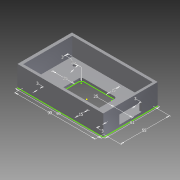
# Autodesk Inventor part: layer line sensor
Saved by Autodesk Inventor 2012 (Build 160160000, 160)
## iProperties
Created: 2012-11-27
Part Number: layer line sensor
Material: Default
Document SubType Name: Modeling
Designer: irwan
Density: 1 g/cm^3
Author: irwan
Autodesk Inventor part; units mm, degrees
ref_plane "YZ Plane" through (0, 0, 0) normal (1, 0, 0) x (0, 1, 0)
ref_plane "XZ Plane" through (0, 0, 0) normal (0, 1, 0) x (-1, 0, 0)
ref_plane "XY Plane" through (0, 0, 0) normal (0, 0, 1) x (1, 0, 0)
sketch "Sketch1" plane through (0, 0, 0) normal (0, 0, 1) x (1, 0, 0)
  line L0 (-50.0201, 33.5227) -> (45.9799, 33.5227)
  line L1 (45.9799, 33.5227) -> (45.9799, -27.4773)
  line L2 (45.9799, -27.4773) -> (-50.0201, -27.4773)
  line L3 (-50.0201, -27.4773) -> (-50.0201, 33.5227)
  line L4 (-50.0201, 33.5227) -> (-50.0201, 30.5227)
  line L5 (-46.6334, 30.5227) -> (43.3666, 30.5227)
  line L6 (43.3666, 30.5227) -> (43.3666, -24.4773)
  line L7 (43.3666, -24.4773) -> (-46.6334, -24.4773)
  line L8 (-46.6334, -24.4773) -> (-46.6334, 30.5227)
  circle A0 centre (-36.6334, 23.0227) radius 1.5
  circle A1 centre (33.3666, 23.0227) radius 1.5
  circle A2 centre (-36.6334, -16.9773) radius 1.5
  circle A3 centre (33.3666, -16.9773) radius 1.5
  line L9 (-18.6334, 15.5227) -> (15.3666, 15.5227)
  line L10 (18.3666, 12.5227) -> (18.3666, -6.4773)
  line L11 (15.3666, -9.4773) -> (-18.6334, -9.4773)
  line L12 (-21.6334, -6.4773) -> (-21.6334, 12.5227)
  arc A4 (-18.6334, 15.5227) -> (-21.6334, 12.5227) centre (-18.6334, 12.5227) ccw
  arc A5 (18.3666, 12.5227) -> (15.3666, 15.5227) centre (15.3666, 12.5227) ccw
  arc A6 (15.3666, -9.4773) -> (18.3666, -6.4773) centre (15.3666, -6.4773) ccw
  arc A7 (-21.6334, -6.4773) -> (-18.6334, -9.4773) centre (-18.6334, -6.4773) ccw
  point P0 (0, 0)
  dimension "d0" = 96
  dimension "d1" = 61
  dimension "d4" = 90
  dimension "d5" = 55
  dimension "d6" = 3
  dimension "d14" = 3
  dimension "d17" = 3
  dimension "d20" = 3
  dimension "d22" = 3
  dimension "d24" = 25
  dimension "d25" = 25
  dimension "d26" = 15
  dimension "d27" = 15
  dimension "d28" = 3
  constraints: 26 end point, 8 centre point, 8 point on circle, 8 tangent, 5 parallel, 5 perpendicular, 3 equal radius, 2 horizontal, 1 point on line
  measures "d0" distance of L1.end L2.end
  measures "d1" distance of L0.end L1.end
  measures "d4" distance of L6.end L7.end
  measures "d5" distance of L5.end L6.end
  measures "d6" distance between parallel lines of L0 L5
  measures "d14" diameter of A0
  measures "d17" diameter of A1
  measures "d20" diameter of A2
  measures "d22" diameter of A3
  measures "d24" distance between parallel lines of L12 L8
  measures "d25" distance between parallel lines of L10 L6
  measures "d26" distance between parallel lines of L9 L5
  measures "d27" distance between parallel lines of L7 L11
  measures "d28" radius of A4
extrude "Extrusion2" add sketch "Sketch1" along normal blind 23 contours L0 L1 L2 L3
extrude "Extrusion3" add sketch "Sketch1" along normal blind 3 contours L5 L6 L7 L8
sketch "Sketch2" plane through (45.9799, -27.4773, 0) normal (1, 0, 0) x (0, 0, -1)
  line L0 (0, 0) -> (-23, 0) projected
  line L1 (0, 0) -> (0, 61) projected
  line L2 (-13, 18) -> (-3, 18)
  line L3 (-3, 18) -> (-3, 43)
  line L4 (-3, 43) -> (-13, 43)
  line L5 (-13, 43) -> (-13, 18)
  point P0 (0, 27.4773)
  dimension "d33" = 10
  dimension "d34" = 25
  dimension "d35" = 3
  dimension "d36" = 18
  constraints: 8 end point, 2 parallel, 1 horizontal, 1 perpendicular
  measures "d33" distance of L4.end L3.end
  measures "d34" distance of L3.end L2.end
  measures "d35" distance between parallel lines of L3 L1
  measures "d36" distance between parallel lines of L2 L0
extrude "Extrusion4" cut sketch "Sketch2" against normal blind 3
body "Solid1"
